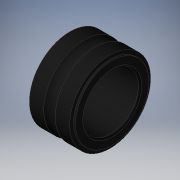
# Autodesk Inventor part: 6000DDU Inner ring
Saved by Autodesk Inventor 2019 (Build 230136000, 136)
## iProperties
Created: 2023-07-21
Part Number: 6000DDU Inner ring
Material: Generic
Catalog Web Link: www.cadenas.de
Description: contact_sealed_type_dd_ddu_IR-NSK
Vendor: NSK_RB
Document SubType Name: Modeling
Designer: psAdmin
Manufacturer: NSK_RB
Mass: 0.664402 g
Surface Area: 7.84888 cm^2
Volume: 0.664402 cm^3
Density: 1 g/cm^3
Appearance: PSOLRGB-128-128-128
Category: PARTsolutions
Company: NSK_RB
Title: 6000DDU Inner ring
Author: Cadenas PARTsolutions
Comments: NSK
PSOL_IDENT_0: {$CADENAS_DATA/23d-libs/nsk_rb/roller_bearings/deep_groove_bb/single_row_dgbb/contact_sealed_type_dd
PSOL_IDENT_1: _ddu_3_ir.prj},199 {VTYP=3D},{NB=6000DDU Inner ring},{LINA=6000DDU Inner ring},{NN=contact_sealed_ty
PSOL_IDENT_2: pe_dd_ddu_IR},{DATE=15.09.2022 00:32:48},{GEOMDATE=18.05.2018 11:36:18},{VERSION=},{LINEID=30},{WBVA
PSOL_IDENT_3: R=},{WBNUMERIC=}  {NB=6000DDU Inner ring},{LINA=6000DDU Inner ring},{KT=DUMMY},{IDNR=},{STAN=Standar
PSOL_IDENT_4: d},{ORDER=6000DDU},{SD=10},{X=10},{DI1=14.57},{DI2=13.2},{SDE1=21.50},{SDE2=23.00},{D=26},{DD=26},{B=
PSOL_IDENT_5: 8},{R=0.3},{CR1=4550},{COR1=1970},{CR2=465},{COR2=201},{FO=12.4},{LG=22000},{A=1.35},{BB=0.87},{DD1=
PSOL_IDENT_6: 24.50},{RO=0.20},{RN=0.3},{DD2=28.7},{F=0.84},{DAM1=12.0},{DA1=13.0},{DA2=24.0},{RA=0.3},{DX=29.4},{
PSOL_IDENT_7: CY=1.9},{MASS=0.018},{SC=1}
NB: 6000DDU Inner ring
NN: contact_sealed_type_dd_ddu_IR
NT: NSK
NBSYN: $ORDER. Inner ring
LINA: 6000DDU Inner ring
CATALOG: NSK Rolling Bearing
STAN: Standard
ORDER: 6000DDU
SD: 10
X: 10
DI1: 14.57
DI2: 13.2
SDE1: 21.5
SDE2: 23
D: 26
DD: 26
B: 8
R: 0.3
CR1: 4550
COR1: 1970
CR2: 465
COR2: 201
FO: 12.4
LG: 22000
A: 1.35
BB: 0.87
DD1: 24.5
RO: 0.2
RN: 0.3
DD2: 28.7
F: 0.84
DAM1: 12
DA1: 13
DA2: 24
RA: 0.3
DX: 29.4
CY: 1.9
MASS: 0.018
SC: 1
SUPPLIER: NSK_RB
ARTICLENO: 6000DDU Inner ring
BOMINFO: 6000DDU Inner ring
CREATOR: CADENAS GmbH
Autodesk Inventor part; units mm, degrees
ref_plane "YZ Plane" through (0, 0, 0) normal (1, 0, 0) x (0, 1, 0)
ref_plane "XZ Plane" through (0, 0, 0) normal (0, 1, 0) x (-1, 0, 0)
ref_plane "XY Plane" through (0, 0, 0) normal (0, 0, 1) x (1, 0, 0)
sketch "Sketch_1" plane through (0, 0, 0) normal (0, 0, 1) x (1, 0, 0)
  line L0 (8, 0) -> (0, 0)
  arc A0 (0, 5.3) -> (0.3, 5) centre (0.3, 5.3) ccw
  line L1 (0.3, 5) -> (7.7, 5)
  arc A1 (7.7, 5) -> (8, 5.3) centre (7.7, 5.3) ccw
  line L2 (8, 5.3) -> (8, 6.6)
  line L3 (8, 6.6) -> (7.632, 6.6)
  line L4 (7.632, 6.6) -> (7.632, 7.285)
  line L5 (7.632, 7.285) -> (5.029, 7.285)
  arc A2 (2.971, 7.285) -> (5.029, 7.285) centre (4, 9) ccw
  line L6 (2.971, 7.285) -> (0.368, 7.285)
  line L7 (0.368, 7.285) -> (0.368, 6.6)
  line L8 (0.368, 6.6) -> (0, 6.6)
  line L9 (0, 6.6) -> (0, 5.3)
  constraints: 20 end point, 6 point on circle, 3 centre point
revolve "Revolution1" add sketch "Sketch_1" angle 360 about axis through (8, 0, 0) along (1, 0, 0)
ref_plane "ip_cst_3_ir_1_1_XY" through (4, 9, 0) normal (-1, 0, 0) x (0, 0, -1)
ref_plane "ip_cst_3_ir_1_1_YZ" through (4, 9, 0) normal (0, 0, -1) x (0, -1, 0)
ref_plane "ip_cst_3_ir_1_1_ZX" through (4, 9, 0) normal (0, -1, 0) x (-1, 0, 0)
ref_plane "ip_cst_3_ir_1_10_XY" through (4, -3.1914, -8.4151) normal (-1, 0, 0) x (0, 0, -1)
ref_plane "ip_cst_3_ir_1_10_YZ" through (4, -3.1914, -8.4151) normal (0, 0, -1) x (0, -1, 0)
ref_plane "ip_cst_3_ir_1_10_ZX" through (4, -3.1914, -8.4151) normal (0, -1, 0) x (-1, 0, 0)
ref_plane "ip_cst_3_ir_1_11_XY" through (4, 1.0848, -8.9344) normal (-1, 0, 0) x (0, 0, -1)
ref_plane "ip_cst_3_ir_1_11_YZ" through (4, 1.0848, -8.9344) normal (0, 0, -1) x (0, -1, 0)
ref_plane "ip_cst_3_ir_1_11_ZX" through (4, 1.0848, -8.9344) normal (0, -1, 0) x (-1, 0, 0)
ref_plane "ip_cst_3_ir_1_12_XY" through (4, 5.1126, -7.4069) normal (-1, 0, 0) x (0, 0, -1)
ref_plane "ip_cst_3_ir_1_12_YZ" through (4, 5.1126, -7.4069) normal (0, 0, -1) x (0, -1, 0)
ref_plane "ip_cst_3_ir_1_12_ZX" through (4, 5.1126, -7.4069) normal (0, -1, 0) x (-1, 0, 0)
ref_plane "ip_cst_3_ir_1_13_XY" through (4, 7.9691, -4.1825) normal (-1, 0, 0) x (0, 0, -1)
ref_plane "ip_cst_3_ir_1_13_YZ" through (4, 7.9691, -4.1825) normal (0, 0, -1) x (0, -1, 0)
ref_plane "ip_cst_3_ir_1_13_ZX" through (4, 7.9691, -4.1825) normal (0, -1, 0) x (-1, 0, 0)
ref_plane "ip_cst_3_ir_1_2_XY" through (4, 7.9691, 4.1825) normal (-1, 0, 0) x (0, 0, -1)
ref_plane "ip_cst_3_ir_1_2_YZ" through (4, 7.9691, 4.1825) normal (0, 0, -1) x (0, -1, 0)
ref_plane "ip_cst_3_ir_1_2_ZX" through (4, 7.9691, 4.1825) normal (0, -1, 0) x (-1, 0, 0)
ref_plane "ip_cst_3_ir_1_3_XY" through (4, 5.1126, 7.4069) normal (-1, 0, 0) x (0, 0, -1)
ref_plane "ip_cst_3_ir_1_3_YZ" through (4, 5.1126, 7.4069) normal (0, 0, -1) x (0, -1, 0)
ref_plane "ip_cst_3_ir_1_3_ZX" through (4, 5.1126, 7.4069) normal (0, -1, 0) x (-1, 0, 0)
ref_plane "ip_cst_3_ir_1_4_XY" through (4, 1.0848, 8.9344) normal (-1, 0, 0) x (0, 0, -1)
ref_plane "ip_cst_3_ir_1_4_YZ" through (4, 1.0848, 8.9344) normal (0, 0, -1) x (0, -1, 0)
ref_plane "ip_cst_3_ir_1_4_ZX" through (4, 1.0848, 8.9344) normal (0, -1, 0) x (-1, 0, 0)
ref_plane "ip_cst_3_ir_1_5_XY" through (4, -3.1914, 8.4151) normal (-1, 0, 0) x (0, 0, -1)
ref_plane "ip_cst_3_ir_1_5_YZ" through (4, -3.1914, 8.4151) normal (0, 0, -1) x (0, -1, 0)
ref_plane "ip_cst_3_ir_1_5_ZX" through (4, -3.1914, 8.4151) normal (0, -1, 0) x (-1, 0, 0)
ref_plane "ip_cst_3_ir_1_6_XY" through (4, -6.7366, 5.9681) normal (-1, 0, 0) x (0, 0, -1)
ref_plane "ip_cst_3_ir_1_6_YZ" through (4, -6.7366, 5.9681) normal (0, 0, -1) x (0, -1, 0)
ref_plane "ip_cst_3_ir_1_6_ZX" through (4, -6.7366, 5.9681) normal (0, -1, 0) x (-1, 0, 0)
ref_plane "ip_cst_3_ir_1_7_XY" through (4, -8.7385, 2.1538) normal (-1, 0, 0) x (0, 0, -1)
ref_plane "ip_cst_3_ir_1_7_YZ" through (4, -8.7385, 2.1538) normal (0, 0, -1) x (0, -1, 0)
ref_plane "ip_cst_3_ir_1_7_ZX" through (4, -8.7385, 2.1538) normal (0, -1, 0) x (-1, 0, 0)
ref_plane "ip_cst_3_ir_1_8_XY" through (4, -8.7385, -2.1538) normal (-1, 0, 0) x (0, 0, -1)
ref_plane "ip_cst_3_ir_1_8_YZ" through (4, -8.7385, -2.1538) normal (0, 0, -1) x (0, -1, 0)
ref_plane "ip_cst_3_ir_1_8_ZX" through (4, -8.7385, -2.1538) normal (0, -1, 0) x (-1, 0, 0)
ref_plane "ip_cst_3_ir_1_9_XY" through (4, -6.7366, -5.9681) normal (-1, 0, 0) x (0, 0, -1)
ref_plane "ip_cst_3_ir_1_9_YZ" through (4, -6.7366, -5.9681) normal (0, 0, -1) x (0, -1, 0)
ref_plane "ip_cst_3_ir_1_9_ZX" through (4, -6.7366, -5.9681) normal (0, -1, 0) x (-1, 0, 0)
ref_plane "ip_cst_3_ir_1a_XY" through (0, 0, 0) normal (1, 0, 0) x (0, 0, -1)
ref_plane "ip_cst_3_ir_1a_YZ" through (0, 0, 0) normal (0, 0, -1) x (0, 1, 0)
ref_plane "ip_cst_3_ir_1a_ZX" through (0, 0, 0) normal (0, 1, 0) x (1, 0, 0)
body "Solid1"
